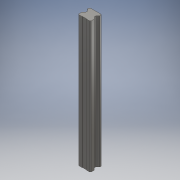
# Autodesk Inventor part: LinearRail
Saved by Autodesk Inventor 2018 (Build 220112000, 112)
## iProperties
Created: 2017-10-19
Part Number: LinearRail
Material: Stainless Steel
Document SubType Name: Modeling
Designer: Bryce Richards
Density: 8 g/cm^3
Appearance: Semi-Polished
Author: Bryce Richards
Autodesk Inventor part; units mm, degrees
ref_plane "YZ Plane" through (0, 0, 0) normal (1, 0, 0) x (0, 1, 0)
ref_plane "XZ Plane" through (0, 0, 0) normal (0, 1, 0) x (-1, 0, 0)
ref_plane "XY Plane" through (0, 0, 0) normal (0, 0, 1) x (1, 0, 0)
sketch "Sketch1" plane through (0, 0, 0) normal (0, 0, 1) x (1, 0, 0)
  line L0 (-7.5, 0) -> (7.5, 0)
  line L1 (0, 0) -> (0, 20) construction
  line L2 (-6.5, 14) -> (6.5, 14)
  line L3 (-7.5, 0) -> (-7.5, 4.6)
  line L4 (7.5, 0) -> (7.5, 4.6)
  line L5 (-5, 7.1) -> (-5, 9)
  line L6 (5, 7.1) -> (5, 9)
  line L7 (-7.5, 11.5) -> (-7.5, 13)
  line L8 (7.5, 11.5) -> (7.5, 13)
  arc A0 (-6.5, 10.5) -> (-7.5, 11.5) centre (-7.9354, 10.0646) ccw
  arc A1 (-7.5, 13) -> (-6.5, 14) centre (-7.9354, 14.4354) ccw
  arc A2 (6.5, 14) -> (7.5, 13) centre (7.9354, 14.4354) ccw
  arc A3 (7.5, 11.5) -> (6.5, 10.5) centre (7.9354, 10.0646) ccw
  line L9 (-7.5, 4.6) -> (-5, 7.1)
  line L10 (7.5, 4.6) -> (5, 7.1)
  line L11 (-6.5, 10.5) -> (-5, 9)
  line L12 (6.5, 10.5) -> (5, 9)
  point P0 (-5, 0)
  point P1 (-5, 8.6667)
  point P2 (5, 0)
  point P3 (5, 8.6667)
  point P4 (7.5, 12.25)
  point P5 (-7.5, 12.25)
  point P6 (0, 14)
  point P7 (-5.75, 6.35)
  point P8 (5.75, 6.35)
  point P9 (0, 10)
  point P10 (0, 10.5)
  dimension "d0" = 15
  dimension "d3" = 14
  dimension "d4" = 4.6
  dimension "d5" = 5
  dimension "d20" = 7.5
  dimension "d21" = 7.5
  dimension "d22" = 1.5
  dimension "d23" = 1.5
  dimension "d25" = 1.5
  dimension "d40" = 15
  dimension "d52" = 45
  dimension "d54" = 1.5
  dimension "d55" = 1
  dimension "d56" = 1
  dimension "d57" = 1
  dimension "d58" = 1
  dimension "d59" = 1
  dimension "d60" = 1
  dimension "d61" = 45
  dimension "d62" = 45
  dimension "d63" = 13
  dimension "d64" = 10
  dimension "d65" = 3.5
  constraints: 26 end point, 8 point on circle, 6 midpoint, 5 parallel, 5 point on line, 4 centre point, 4 symmetric about line, 2 vertical, 1 coincident, 1 horizontal, 1 vertical alignment
  measures "d0" distance of L0.start L0.end
  measures "d3" distance between parallel lines of L0 L2
  measures "d4" distance of L0.start L3.end
  measures "d5" distance between parallel lines of L1 L5
  measures "d20" distance between parallel lines of L1 L7
  measures "d21" distance between parallel lines of L1 L8
  measures "d22" radius of A1
  measures "d23" radius of A0
  measures "d25" radius of A3
  measures "d40" distance of L8.end L7.end
  measures "d52" angle of L5 L9
  measures "d54" radius of A2
  measures "d55" horizontal distance of L2.end L8.end
  measures "d56" horizontal distance of L8.end L2.end
  measures "d57" horizontal distance of L7.end L2.start
  measures "d58" horizontal distance of L11.start L7.start
  measures "d59" horizontal distance of L7.start L11.start
  measures "d60" horizontal distance of L12.start L8.start
  measures "d61" angle of L5 L11
  measures "d62" angle of L6 L12
  measures "d63" distance of L12.start L11.start
  measures "d64" distance of L6.end L5.end
  measures "d65" distance from line of L2 L11.start
extrude "Extrusion1" add sketch "Sketch1" along normal blind 160
chamfer "Chamfer1" distance 1 angle 45 2 edges at (-7.5, 0, 80) (7.5, 0, 80)
sketch "Sketch3" plane through (0, 0, 160) normal (0, 0, 1) x (1, 0, 0)
  line L0 (-6.5, 0) -> (6.5, 0) construction
  line L1 (0, 0) -> (0, 0.3) construction
  line L2 (-2.25, 0) -> (-2.25, 0.3)
  line L3 (2.25, 0) -> (2.25, 0.3)
  line L4 (-2.25, 0.3) -> (2.25, 0.3)
  line L5 (-2.25, 0) -> (2.25, 0)
  line L6 (-6.5, 0) -> (6.5, 0) construction
  dimension "d71" = 0.3
  dimension "d72" = 2.25
  dimension "d73" = 0.3
  dimension "d74" = 0
  constraints: 10 end point, 2 parallel, 2 symmetric about line, 1 collinear, 1 horizontal, 1 vertical
  measures "d71" distance of L1.start L1.end
  measures "d72" distance between parallel lines of L1 L2
  measures "d73" distance between parallel lines of L0 L4
  measures "d74" distance between parallel lines of L5 L0
extrude "Extrusion2" cut sketch "Sketch3" against normal through all
chamfer "Chamfer2" distance 0.3 angle 45 2 edges at (-2.25, 0, 80) (2.25, 0, 80)
body "Solid1"
